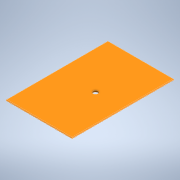
# Autodesk Inventor part: BaseExtrusion
Saved by Autodesk Inventor 2021 (Build 250183000, 183)
## iProperties
Created: 2021-04-17
Part Number: BaseExtrusion
Material: Generic
Document SubType Name: Modeling
Designer: GABRIEL LOL
Density: 1 g/cm^3
Appearance: Orange
Author: GABRIEL LOL
Autodesk Inventor part; units mm, degrees
ref_plane "YZ Plane" through (0, 0, 0) normal (1, 0, 0) x (0, 1, 0)
ref_plane "XZ Plane" through (0, 0, 0) normal (0, 1, 0) x (-1, 0, 0)
ref_plane "XY Plane" through (0, 0, 0) normal (0, 0, 1) x (1, 0, 0)
sketch "Sketch1" plane through (0, 0, 0) normal (0, 1, 0) x (-1, 0, 0)
  line L0 (138, 213) -> (-138, 213)
  line L1 (-138, 213) -> (-138, -213)
  line L2 (-138, -213) -> (138, -213)
  line L3 (138, -213) -> (138, 213)
  line L4 (138, 213) -> (-138, -213) construction
  line L5 (-138, 213) -> (138, -213) construction
  line L6 (0, 0) -> (-23, 0) construction
  circle A0 centre (-23, 0) radius 10
  dimension "d0" = 276
  dimension "d1" = 426
  dimension "d2" = 23
  dimension "d3" = 20
  constraints: 14 end point, 2 horizontal, 2 midpoint, 2 parallel, 1 centre point, 1 coincident, 1 perpendicular
  measures "d0" distance of L2.end L1.end
  measures "d1" distance of L1.end L0.end
  measures "d2" distance of L6.start L6.end
  measures "d3" diameter of A0
extrude "Extrusion1" add sketch "Sketch1" along normal blind 6
fillet "Fillet1" radius 2 8 edges at (0, 6, 213) (138, 6, 0) (-138, 6, 0) (0, 6, -213) (138, 0, 0) (0, 0, 213) (0, 0, -213) (-138, 0, 0)
body "Solid1"
